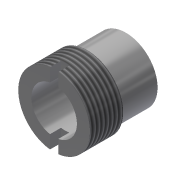
# Autodesk Inventor part: Collar
Saved by Autodesk Inventor 2022 Beta2 (Build 260130000, 130) ContinuousBuild 0
## iProperties
Created: 2006-01-18
Part Number: Collar
Document SubType Name: Modeling
Designer: PMiller
Material: Steel, Mild
Density: 7.86 g/cm^3
Appearance: Steel
Author: PMiller
Autodesk Inventor part; units mm, degrees
ref_plane "YZ Plane" through (0, 0, 0) normal (1, 0, 0) x (0, 1, 0)
ref_plane "XZ Plane" through (0, 0, 0) normal (0, 1, 0) x (-1, 0, 0)
ref_plane "XY Plane" through (0, 0, 0) normal (0, 0, 1) x (1, 0, 0)
sketch "Sketch1" plane through (0, 0, 0) normal (0, 0, 1) x (1, 0, 0)
  circle A0 centre (0, 0) radius 6.5484
  circle A1 centre (0, 0) radius 10.3188
  dimension "d0" = 20.6375
  dimension "d1" = 13.0969
  constraints: 2 centre point, 2 coincident
  measures "d0" diameter of A1
  measures "d1" diameter of A0
extrude "Extrusion1" add sketch "Sketch1" against normal blind 9.525
sketch "Sketch2" plane through (0, 0, -9.525) normal (0, 0, -1) x (-1, 0, 0)
  circle A0 centre (0, 0) radius 6.5484 projected
  circle A1 centre (0, 0) radius 10.3188 projected
  circle A2 centre (0, 0) radius 9.1281
  dimension "d4" = 18.2563
  constraints: 1 centre point, 1 coincident
  measures "d4" diameter of A2
extrude "Extrusion2" add sketch "Sketch2" along normal blind 11.1125 contours A2
sketch "Sketch3" plane through (0, 0, 0) normal (0, 1, 0) x (-1, 0, 0)
  line L0 (-10.3188, 0) -> (10.3188, 0) projected
  line L1 (-1.1906, 0) -> (-1.1906, -3.175)
  line L2 (-1.1906, -3.175) -> (1.1906, -3.175)
  line L3 (1.1906, -3.175) -> (1.1906, 0)
  point P0 (0, -3.175)
  point P1 (0, 0)
  dimension "d7" = 3.175
  dimension "d8" = 2.3813
  constraints: 6 end point, 3 perpendicular, 2 midpoint, 2 point on line, 1 vertical alignment
  measures "d7" distance of L1.start L1.end
  measures "d8" distance of L1.end L2.end
extrude "Extrusion3" cut sketch "Sketch3" along normal through all both and the other way through all
thread "Thread1" size "13/16-20 UNEF" class "3A" standard "ANSI Unified Screw Threads" full length
body "Solid1"
